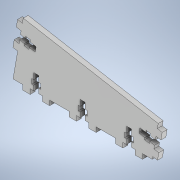
# Autodesk Inventor part: tc_support_down
Saved by Autodesk Inventor 2020.1 (Build 241239000, 239)
## iProperties
Created: 2019-07-16
Part Number: tc_support_down
Material: Acier inoxydable
Document SubType Name: Modeling
Designer: Thibault
Density: 8 g/cm^3
Appearance: Semi-poli
extra_height_front: 11,000 mm
extra_height_back: 1,108 mm
tc_base_support_dist: 56,100 mm
tc_anchor_dist: 19,000 mm
Author: Thibault
Autodesk Inventor part; units mm, degrees
ref_plane "YZ Plane" through (0, 0, 0) normal (1, 0, 0) x (0, 1, 0)
ref_plane "XZ Plane" through (0, 0, 0) normal (0, 1, 0) x (-1, 0, 0)
ref_plane "XY Plane" through (0, 0, 0) normal (0, 0, 1) x (1, 0, 0)
sketch "Anchor (screw side)" plane through (0, 0, 0) normal (0, 0, 1) x (1, 0, 0)
  circle A0 centre (93.7216, 50.3096) radius 1.05
  line L0 (91.2716, 51.3596) -> (88.1716, 51.3596)
  line L1 (88.1716, 51.3596) -> (88.1716, 49.2596)
  line L2 (88.1716, 49.2596) -> (91.2716, 49.2596)
  line L3 (91.2716, 49.2596) -> (91.2716, 51.3596)
  line L4 (99.2716, 51.3596) -> (96.1716, 51.3596)
  line L5 (96.1716, 51.3596) -> (96.1716, 49.2596)
  line L6 (96.1716, 49.2596) -> (99.2716, 49.2596)
  line L7 (99.2716, 49.2596) -> (99.2716, 51.3596)
  line L8 (91.2716, 51.3596) -> (96.1716, 49.2596) construction
  line L9 (96.1716, 51.3596) -> (91.2716, 49.2596) construction
  line L10 (86.1716, 53.3596) -> (101.2716, 53.3596) construction
  line L11 (101.2716, 53.3596) -> (101.2716, 47.2596) construction
  line L12 (101.2716, 47.2596) -> (86.1716, 47.2596) construction
  line L13 (86.1716, 47.2596) -> (86.1716, 53.3596) construction
  point P0 (103.5798, 50.1132)
  dimension "d27" = 2.1
  dimension "d28" = 3.1
  dimension "d29" = 2.1
  dimension "d32" = 4.9
  dimension "d34" = 2
  dimension "d35" = 2
  dimension "d36" = 2
  dimension "d37" = 2
  measures "d27" diameter of A0
  measures "d28" distance of L2.end L1.end
  measures "d29" distance of L1.end L0.end
  measures "d32" distance between parallel lines of L5 L3
  measures "d34" distance between parallel lines of L0 L10
  measures "d35" distance between parallel lines of L12 L2
  measures "d36" distance between parallel lines of L11 L7
  measures "d37" distance between parallel lines of L13 L1
sketch "Anchor (nut side)" plane through (0, 0, 0) normal (0, 0, 1) x (1, 0, 0)
  line L0 (10, 0) -> (8.55, 0)
  line L1 (8.55, 0) -> (8.55, -2)
  line L2 (8.55, -2) -> (9.35, -2)
  line L3 (9.35, -2) -> (9.35, -4)
  line L4 (5.65, -4) -> (5.65, -2)
  line L5 (5.65, -2) -> (6.45, -2)
  line L6 (6.45, -2) -> (6.45, 0)
  line L7 (6.45, 0) -> (5, 0)
  line L8 (2, 0) -> (2, 2)
  line L9 (2, 0) -> (3, 0) construction
  line L10 (2, 2) -> (5, 2)
  line L11 (5, 2) -> (5, 0)
  line L12 (10, 0) -> (10, 2)
  line L13 (10, 2) -> (13, 2)
  line L14 (13, 2) -> (13, 0)
  line L15 (0, 0) -> (2, 0)
  line L16 (13, 0) -> (15, 0)
  line L17 (5.65, -4) -> (6.45, -4)
  line L18 (9.35, -4) -> (8.55, -4)
  line L19 (6.45, -4) -> (6.45, -6.25)
  line L20 (8.55, -4) -> (8.55, -6.25)
  line L21 (6.7, -6.5) -> (7.5, -6.5)
  arc A0 (6.45, -6.25) -> (6.7, -6.5) centre (6.7, -6.25) ccw
  arc A1 (8.3, -6.5) -> (8.55, -6.25) centre (8.3, -6.25) ccw
  line L22 (7.5, -6.5) -> (8.3, -6.5)
  line L23 (7.5, -3.8983) -> (7.5, -9.959) construction
  point P0 (9.1321, -0.6227)
  point P1 (6.45, -6.5)
  point P2 (8.55, -6.5)
  dimension "d3" = 2
  dimension "d7" = 5
  dimension "d10" = 1.45
  dimension "d11" = 2
  dimension "d12" = 0.8
  dimension "d13" = 2
  dimension "d14" = 0.8
  dimension "d15" = 2.1
  dimension "d18" = 2
  dimension "d19" = 0.8
  dimension "d20" = 0.8
  dimension "d21" = 2.5
  dimension "d22" = 2.5
  dimension "d23" = 2.1
  dimension "d38" = 2
  dimension "d39" = 0.25
  dimension "d120" = 3
  measures "d3" distance of point (0, 0) L8.start
  measures "d7" distance of L7.end L0.start
  measures "d10" distance of L0.start L0.end
  measures "d11" distance of L0.end L1.end
  measures "d12" distance of L1.end L2.end
  measures "d13" distance of L2.end L3.end
  measures "d14" distance of L4.end L5.end
  measures "d15" distance of L6.end L0.end
  measures "d18" distance of L14.end point (15, 0)
  measures "d19" distance of L4.start L17.end
  measures "d20" distance of L3.end L18.end
  measures "d21" distance of L17.end point (6.45, -6.5)
  measures "d22" distance of L18.end point (8.55, -6.5)
  measures "d23" distance of L17.end L18.end
  measures "d38" distance of the line from the sketch origin of L10
  measures "d39" radius of A0
  measures "d120" distance of L8.end L10.end
derived "shared_parameters.ipt"
sketch "Esquisse2" plane through (0, 0, 0) normal (0, 0, 1) x (1, 0, 0)
  line L0 (-1.0235, 16.109) -> (2.9765, 16.109)
  line L1 (17.9765, 16.109) -> (21.9765, 16.109)
  line L2 (-16.0235, 16.109) -> (-18.0062, 16.109)
  line L3 (36.9765, 16.109) -> (38.9592, 16.109)
  line L4 (-18.0062, 16.109) -> (-16.4434, 24.9722)
  line L5 (-13.8387, 39.7443) -> (41.409, 30.0027)
  line L6 (38.8043, 15.2306) -> (38.9592, 16.109)
  line L7 (-11.0235, 16.109) -> (-9.5735, 16.109)
  line L8 (-9.5735, 16.109) -> (-9.5735, 18.109)
  line L9 (-9.5735, 18.109) -> (-10.3735, 18.109)
  line L10 (-10.3735, 18.109) -> (-10.3735, 20.109)
  line L11 (-6.6735, 20.109) -> (-6.6735, 18.109)
  line L12 (-6.6735, 18.109) -> (-7.4735, 18.109)
  line L13 (-7.4735, 18.109) -> (-7.4735, 16.109)
  line L14 (-7.4735, 16.109) -> (-6.0235, 16.109)
  line L15 (-3.0235, 16.109) -> (-3.0235, 14.109)
  line L16 (-3.0235, 16.109) -> (-4.0235, 16.109) construction
  line L17 (-3.0235, 14.109) -> (-6.0235, 14.109)
  line L18 (-6.0235, 14.109) -> (-6.0235, 16.109)
  line L19 (-11.0235, 16.109) -> (-11.0235, 14.109)
  line L20 (-11.0235, 14.109) -> (-14.0235, 14.109)
  line L21 (-14.0235, 14.109) -> (-14.0235, 16.109)
  line L22 (-1.0235, 16.109) -> (-3.0235, 16.109)
  line L23 (-14.0235, 16.109) -> (-16.0235, 16.109)
  line L24 (-6.6735, 20.109) -> (-7.4735, 20.109)
  line L25 (-10.3735, 20.109) -> (-9.5735, 20.109)
  line L26 (-7.4735, 20.109) -> (-7.4735, 22.359)
  line L27 (-9.5735, 20.109) -> (-9.5735, 22.359)
  line L28 (-7.7235, 22.609) -> (-8.5235, 22.609)
  arc A0 (-7.4735, 22.359) -> (-7.7235, 22.609) centre (-7.7235, 22.359) ccw
  arc A1 (-9.3235, 22.609) -> (-9.5735, 22.359) centre (-9.3235, 22.359) ccw
  line L29 (-8.5235, 22.609) -> (-9.3235, 22.609)
  line L30 (-8.5235, 20.0072) -> (-8.5235, 26.068) construction
  line L31 (7.9765, 16.109) -> (9.4265, 16.109)
  line L32 (9.4265, 16.109) -> (9.4265, 18.109)
  line L33 (9.4265, 18.109) -> (8.6265, 18.109)
  line L34 (8.6265, 18.109) -> (8.6265, 20.109)
  line L35 (12.3265, 20.109) -> (12.3265, 18.109)
  line L36 (12.3265, 18.109) -> (11.5265, 18.109)
  line L37 (11.5265, 18.109) -> (11.5265, 16.109)
  line L38 (11.5265, 16.109) -> (12.9765, 16.109)
  line L39 (15.9765, 16.109) -> (15.9765, 14.109)
  line L40 (15.9765, 16.109) -> (14.9765, 16.109) construction
  line L41 (15.9765, 14.109) -> (12.9765, 14.109)
  line L42 (12.9765, 14.109) -> (12.9765, 16.109)
  line L43 (7.9765, 16.109) -> (7.9765, 14.109)
  line L44 (7.9765, 14.109) -> (4.9765, 14.109)
  line L45 (4.9765, 14.109) -> (4.9765, 16.109)
  line L46 (17.9765, 16.109) -> (15.9765, 16.109)
  line L47 (4.9765, 16.109) -> (2.9765, 16.109)
  line L48 (12.3265, 20.109) -> (11.5265, 20.109)
  line L49 (8.6265, 20.109) -> (9.4265, 20.109)
  line L50 (11.5265, 20.109) -> (11.5265, 22.359)
  line L51 (9.4265, 20.109) -> (9.4265, 22.359)
  line L52 (11.2765, 22.609) -> (10.4765, 22.609)
  arc A2 (11.5265, 22.359) -> (11.2765, 22.609) centre (11.2765, 22.359) ccw
  arc A3 (9.6765, 22.609) -> (9.4265, 22.359) centre (9.6765, 22.359) ccw
  line L53 (10.4765, 22.609) -> (9.6765, 22.609)
  line L54 (10.4765, 20.0072) -> (10.4765, 26.068) construction
  line L55 (26.9765, 16.109) -> (28.4265, 16.109)
  line L56 (28.4265, 16.109) -> (28.4265, 18.109)
  line L57 (28.4265, 18.109) -> (27.6265, 18.109)
  line L58 (27.6265, 18.109) -> (27.6265, 20.109)
  line L59 (31.3265, 20.109) -> (31.3265, 18.109)
  line L60 (31.3265, 18.109) -> (30.5265, 18.109)
  line L61 (30.5265, 18.109) -> (30.5265, 16.109)
  line L62 (30.5265, 16.109) -> (31.9765, 16.109)
  line L63 (34.9765, 16.109) -> (34.9765, 14.109)
  line L64 (34.9765, 16.109) -> (33.9765, 16.109) construction
  line L65 (34.9765, 14.109) -> (31.9765, 14.109)
  line L66 (31.9765, 14.109) -> (31.9765, 16.109)
  line L67 (26.9765, 16.109) -> (26.9765, 14.109)
  line L68 (26.9765, 14.109) -> (23.9765, 14.109)
  line L69 (23.9765, 14.109) -> (23.9765, 16.109)
  line L70 (36.9765, 16.109) -> (34.9765, 16.109)
  line L71 (23.9765, 16.109) -> (21.9765, 16.109)
  line L72 (31.3265, 20.109) -> (30.5265, 20.109)
  line L73 (27.6265, 20.109) -> (28.4265, 20.109)
  line L74 (30.5265, 20.109) -> (30.5265, 22.359)
  line L75 (28.4265, 20.109) -> (28.4265, 22.359)
  line L76 (30.2765, 22.609) -> (29.4765, 22.609)
  arc A4 (30.5265, 22.359) -> (30.2765, 22.609) centre (30.2765, 22.359) ccw
  arc A5 (28.6765, 22.609) -> (28.4265, 22.359) centre (28.6765, 22.359) ccw
  line L77 (29.4765, 22.609) -> (28.6765, 22.609)
  line L78 (29.4765, 20.0072) -> (29.4765, 26.068) construction
  line L79 (-14.7069, 34.8203) -> (-14.9587, 33.3923)
  line L80 (-14.9587, 33.3923) -> (-12.9891, 33.045)
  line L81 (-12.9891, 33.045) -> (-12.8502, 33.8329)
  line L82 (-12.8502, 33.8329) -> (-10.8806, 33.4856)
  line L83 (-11.5231, 29.8418) -> (-13.4927, 30.1891)
  line L84 (-13.4927, 30.1891) -> (-13.3538, 30.9769)
  line L85 (-13.3538, 30.9769) -> (-15.3234, 31.3242)
  line L86 (-15.3234, 31.3242) -> (-15.5752, 29.8963)
  line L87 (-16.0961, 26.9418) -> (-18.0657, 27.2891)
  line L88 (-16.0961, 26.9418) -> (-15.9225, 27.9266) construction
  line L89 (-18.0657, 27.2891) -> (-17.5448, 30.2436)
  line L90 (-17.5448, 30.2436) -> (-15.5752, 29.8963)
  line L91 (-14.7069, 34.8203) -> (-16.6765, 35.1676)
  line L92 (-16.6765, 35.1676) -> (-16.1556, 38.122)
  line L93 (-16.1556, 38.122) -> (-14.186, 37.7747)
  line L94 (-16.4434, 24.9722) -> (-16.0961, 26.9418)
  line L95 (-14.186, 37.7747) -> (-13.8387, 39.7443)
  line L96 (-11.5231, 29.8418) -> (-11.3841, 30.6296)
  line L97 (-10.8806, 33.4856) -> (-11.0195, 32.6977)
  line L98 (-11.3841, 30.6296) -> (-9.1683, 30.2389)
  line L99 (-11.0195, 32.6977) -> (-8.8037, 32.307)
  line L100 (-8.8787, 30.4417) -> (-8.7398, 31.2296)
  arc A6 (-9.1683, 30.2389) -> (-8.8787, 30.4417) centre (-9.1249, 30.4851) ccw
  arc A7 (-8.6009, 32.0174) -> (-8.8037, 32.307) centre (-8.8471, 32.0608) ccw
  line L101 (-8.7398, 31.2296) -> (-8.6009, 32.0174)
  line L102 (-11.302, 31.6814) -> (-5.3333, 30.6289) construction
  line L103 (39.6726, 20.1546) -> (39.9243, 21.5826)
  line L104 (39.9243, 21.5826) -> (37.9547, 21.9299)
  line L105 (37.9547, 21.9299) -> (37.8158, 21.142)
  line L106 (37.8158, 21.142) -> (35.8462, 21.4893)
  line L107 (36.4887, 25.1331) -> (38.4583, 24.7858)
  line L108 (38.4583, 24.7858) -> (38.3194, 23.998)
  line L109 (38.3194, 23.998) -> (40.289, 23.6507)
  line L110 (40.289, 23.6507) -> (40.5408, 25.0786)
  line L111 (41.0617, 28.0331) -> (43.0314, 27.6858)
  line L112 (41.0617, 28.0331) -> (40.8881, 27.0483) construction
  line L113 (43.0314, 27.6858) -> (42.5104, 24.7313)
  line L114 (42.5104, 24.7313) -> (40.5408, 25.0786)
  line L115 (39.6726, 20.1546) -> (41.6422, 19.8073)
  line L116 (41.6422, 19.8073) -> (41.1212, 16.8529)
  line L117 (41.1212, 16.8529) -> (39.1516, 17.2002)
  line L118 (41.409, 30.0027) -> (41.0617, 28.0331)
  line L119 (39.1516, 17.2002) -> (38.8043, 15.2306)
  line L120 (36.4887, 25.1331) -> (36.3498, 24.3453)
  line L121 (35.8462, 21.4893) -> (35.9851, 22.2772)
  line L122 (36.3498, 24.3453) -> (34.134, 24.736)
  line L123 (35.9851, 22.2772) -> (33.7693, 22.6679)
  line L124 (33.8443, 24.5332) -> (33.7054, 23.7453)
  arc A8 (34.134, 24.736) -> (33.8443, 24.5332) centre (34.0905, 24.4898) ccw
  arc A9 (33.5665, 22.9575) -> (33.7693, 22.6679) centre (33.8127, 22.9141) ccw
  line L125 (33.7054, 23.7453) -> (33.5665, 22.9575)
  line L126 (36.2676, 23.2935) -> (30.299, 24.346) construction
  point P0 (0, 0)
  point P1 (-13.8387, 39.7443)
  point P2 (-17.8871, 8.2607)
  point P3 (38.6612, 14.1706)
  point P4 (-17.9917, 8.6071)
  dimension "d1" = 8
  dimension "d2" = 8
  dimension "tc_anchor_dist" = 19
  dimension "height" = 24
  dimension "d41" = 56.1
  dimension "d44" = 80
  dimension "extra_height_front" = 11
  dimension "extra_height_back" = 1.1081
  constraints: 14 end point, 5 horizontal, 1 collinear, 14 other
  measures "d41" distance of L5.end L5.start
  measures "d44" angle of L2 L4
extrude "Extrusion1" add sketch "Esquisse2" along normal blind 2
equation "\"d41\" = tc_base_support_dist"
equation "\"d31\" = sheet_thickness"
equation "\"tc_base_support_dist\" = 56.1"
equation "\"sheet_thickness\" = 2"
